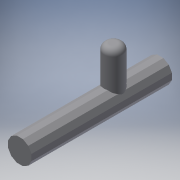
# Autodesk Inventor part: vexCamPost10
Saved by Autodesk Inventor 2016 SP1 (Build 200210100, 210)
## iProperties
Created: 2015-10-16
Part Number: vexCamPost10
Material: Generic
Document SubType Name: Modeling
Designer: steele
Density: 1 g/cm^3
Appearance: Default
Author: steele
Autodesk Inventor part; units mm, degrees
ref_plane "YZ Plane" through (0, 0, 0) normal (1, 0, 0) x (0, 1, 0)
ref_plane "XZ Plane" through (0, 0, 0) normal (0, 1, 0) x (-1, 0, 0)
ref_plane "XY Plane" through (0, 0, 0) normal (0, 0, 1) x (1, 0, 0)
sketch "Sketch1" plane through (0, 0, 0) normal (0, 0, 1) x (1, 0, 0)
  line L0 (3.175, 0.8507) -> (3.175, -0.8507)
  line L1 (3.175, -0.8507) -> (2.3243, -2.3243)
  line L2 (2.3243, -2.3243) -> (0.8507, -3.175)
  line L3 (0.8507, -3.175) -> (-0.8507, -3.175)
  line L4 (-0.8507, -3.175) -> (-2.3243, -2.3243)
  line L5 (-2.3243, -2.3243) -> (-3.175, -0.8507)
  line L6 (-3.175, -0.8507) -> (-3.175, 0.8507)
  line L7 (-3.175, 0.8507) -> (-2.3243, 2.3243)
  line L8 (-2.3243, 2.3243) -> (-0.8507, 3.175)
  line L9 (-0.8507, 3.175) -> (0.8507, 3.175)
  line L10 (0.8507, 3.175) -> (2.3243, 2.3243)
  line L11 (2.3243, 2.3243) -> (3.175, 0.8507)
  line L12 (0, 0) -> (0, 3.175) construction
  dimension "d9" = 6.35
  constraints: 26 end point, 1 parallel, 1 vertical, 25 other
  measures "d9" distance between parallel lines of L0 L6
extrude "Extrusion1" add sketch "Sketch1" along normal blind 25.4 and the other way blind 25.4
sketch "Sketch2" plane through (0, 0, 0) normal (0, 1, 0) x (-1, 0, 0)
  circle A0 centre (0, 0) radius 2.54
  dimension "diamCamSlot" = 5.08
  constraints: 1 centre point, 1 coincident
  measures "diamCamSlot" diameter of A0
extrude "Extrusion2" add sketch "Sketch2" along normal blind 12.7
fillet "Fillet1" radius 1.5875 1 edges at (2.54, 12.7, 0)
equation "\"d9\" = camDiam"
equation "\"camDiam\" = 6.35"
body "Solid1"
